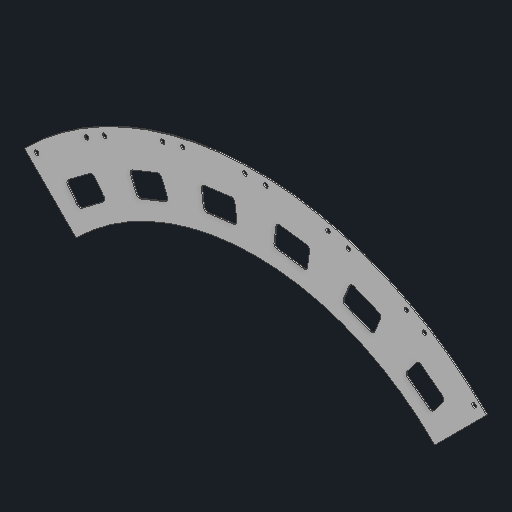
# Autodesk Inventor part: DMF 2.1 01 43 Gear rim 3
Saved by Autodesk Inventor 2026.2 (Build 302298010, 298A)
## iProperties
Created: 2024-04-30
Part Number: DMF 2.1 01 43 Gear rim 3
Material: Generic
Document SubType Name: Sheet Metal
Designer: admin
Stock Number: Барабан_Сектор_Усилителя
Density: 1 g/cm^3
Sheet Metal Rule: Default
Sheet Metal Width: 0,000 mm
Sheet Metal Length: 0,000 mm
Sheet Metal Area: 0,000 mm^2
Appearance: Default
Author: pokla
Autodesk Inventor part; units mm, degrees
ref_plane "YZ Plane" through (0, 0, 0) normal (1, 0, 0) x (0, 1, 0)
ref_plane "XZ Plane" through (0, 0, 0) normal (0, 1, 0) x (-1, 0, 0)
ref_plane "XY Plane" through (0, 0, 0) normal (0, 0, 1) x (1, 0, 0)
sketch "Sketch1" plane through (0, 0, 0) normal (0, 0, 1) x (1, 0, 0)
  circle A0 centre (0, 0) radius 450
  circle A1 centre (0, 0) radius 580
  line L0 (0, 0) -> (-410.1219, 410.1219)
  line L1 (0, 0) -> (0, 580)
  line L2 (0, 0) -> (410.1219, 410.1219)
  point P0 (-318.1981, 318.1981)
  point P1 (318.1981, 318.1981)
  dimension "d30" = 90
  dimension "d31" = 1160
  dimension "d32" = 900
  measures "d30" angle of L2 L0
  measures "d31" diameter of A1
  measures "d32" diameter of A0
extrude "Plate1" add sketch "Sketch1" against normal blind 2 contours A0 L1 A1 L2 | L0 A1 L1 A0
sketch "Sketch3" plane through (0, 0, -2) normal (0, 0, -1) x (-1, 0, 0)
  arc A0 (318.1981, 318.1981) -> (-318.1981, 318.1981) centre (0, 0) ccw projected
  line L0 (410.1219, 410.1219) -> (318.1981, 318.1981) projected
  arc A1 (410.1219, 410.1219) -> (-410.1219, 410.1219) centre (0, 0) ccw projected
  line L1 (-318.1981, 318.1981) -> (-410.1219, 410.1219) projected
  line L2 (-300.9075, 399.3178) -> (0, 0) construction
  line L3 (-336.9029, 397.236) -> (-312.8303, 365.2906)
  line L4 (-312.8303, 365.2906) -> (-264.9121, 401.3995)
  line L5 (-264.9121, 401.3995) -> (-288.9847, 433.3449)
  line L6 (-288.9847, 433.3449) -> (-336.9029, 397.236)
  line L7 (-336.9029, 397.236) -> (-264.9121, 401.3995) construction
  line L8 (-312.8303, 365.2906) -> (-288.9847, 433.3449) construction
  line L9 (0, 0) -> (0, 450) construction
  circle A2 centre (0, 0) radius 500 construction
  point P0 (-288.8712, 383.345)
  dimension "d57" = 1000
  dimension "d53" = 37
  dimension "d55" = 60
  dimension "d56" = 40
  dimension "d58" = 8
  constraints: 16 end point, 3 midpoint, 2 parallel, 1 coincident, 1 perpendicular, 1 point on circle, 1 point on line, 3 other
  measures "d53" angle of L2 L9
  measures "d55" distance of L5.end L3.start
  measures "d56" distance of L4.end L5.end
  measures "d58" angle of L1 L3
extrude "Cut1" cut sketch "Sketch3" against normal blind 2 contours L6 L5 L4 L3
sketch "Sketch2" plane through (0, 0, 0) normal (0, 0, 1) x (1, 0, 0)
  circle A0 centre (0, 0) radius 567.5
  arc A1 (410.1219, 410.1219) -> (-410.1219, 410.1219) centre (0, 0) ccw projected
  line L0 (0, 0) -> (410.1219, 410.1219) construction
  line L1 (0, 0) -> (387.9386, 414.1979) construction
  line L2 (299.6785, 481.9222) -> (0, 0) construction
  line L3 (0, 0) -> (0, 567.5) construction
  line L4 (0, 0) -> (18.5681, 567.1962) construction
  line L5 (0, 0) -> (128.8658, 552.6752) construction
  line L6 (0, 0) -> (267.5176, 500.4903) construction
  line L7 (0, 0) -> (164.7366, 543.0636) construction
  dimension "d34" = 1135
  dimension "d35" = 1.875
  dimension "d36" = 11.25
  dimension "d44" = 1.875
  dimension "d45" = 11.25
  dimension "d49" = 3.75
  dimension "d50" = 11.25
  constraints: 16 end point, 3 coincident, 1 vertical, 9 other
  measures "d35" angle of L0 L1
  measures "d36" angle of L1 L2
  measures "d44" angle of L4 L3
  measures "d45" angle of L5 L4
  measures "d49" angle of L2 L6
  measures "d50" angle of L6 L7
hole "Hole1" at (387.9386, 414.1979, 0) at (299.6785, 481.9222, 0) at (128.8658, 552.6752, 0) at (18.5681, 567.1962, 0) at (267.5176, 500.4903, 0) at (164.7366, 543.0636, 0) direction (0, 0, -1) diameter 8 end through all
pattern_circular "Circular Pattern1" count 2 over 45 about axis through (0, 0, -10) along (0, 0, 1) of "Hole1"
fillet "Corner Round1" radius 6 4 edges at (336.9029, 397.236, -1) (312.8303, 365.2906, -1) (288.9847, 433.3449, -1) (264.9121, 401.3995, -1)
pattern_circular "Circular Pattern2" count 6 over 74 about axis through (0, 0, 0) along (0, 0, 1) of "Cut1", "Corner Round1"
equation "\"d31\" = Колесо_диам1_ручья_внеш"
equation "\"d59\" = Thickness"
equation "\"d44\" = d35"
equation "\"d45\" = d36"
equation "\"d49\" = 2 * d35"
equation "\"d50\" = d36"
equation "\"d42\" = Thickness"
equation "\"d15\" = Thickness"
equation "\"BendRadius\" = Thickness"
equation "\"BendReliefWidth\" = Thickness"
equation "\"BendReliefDepth\" = 0.5 * Thickness"
equation "\"CornerReliefSize\" = 4 * Thickness"
equation "\"MinimumRemnant\" = 2 * Thickness"
equation "\"TransitionRadius\" = BendRadius"
equation "\"JacobiRadiusSize\" = BendRadius"
equation "\"GapSize\" = Thickness"
equation "\"Колесо_диам1_ручья_внеш\" = 1160"
equation "\"Thickness\" = 2"
body "Solid1"
